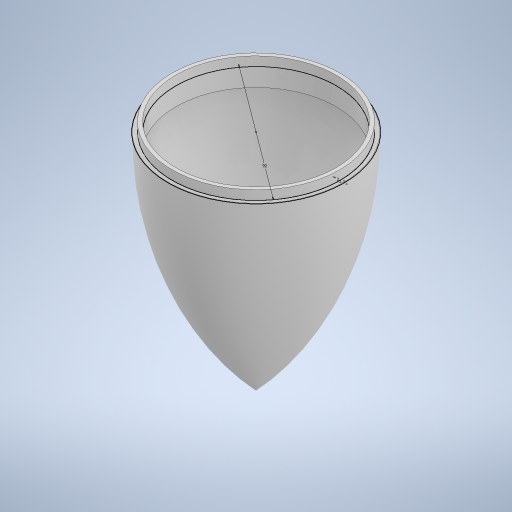
# Autodesk Inventor part: final탄두뚜껑1
Saved by Autodesk Inventor 2023 (Build 270158000, 158)
## iProperties
Created: 2023-10-31
Part Number: final탄두뚜껑1
Material: 일반
Document SubType Name: Modeling
Designer: rlatk
Density: 1 g/cm^3
Appearance: 기본값
Author: rlatk
Autodesk Inventor part; units mm, degrees
ref_plane "YZ Plane" through (0, 0, 0) normal (1, 0, 0) x (0, 1, 0)
ref_plane "XZ Plane" through (0, 0, 0) normal (0, 1, 0) x (-1, 0, 0)
ref_plane "XY Plane" through (0, 0, 0) normal (0, 0, 1) x (1, 0, 0)
sketch "스케치1" plane through (0, 0, 0) normal (0, 1, 0) x (-1, 0, 0)
  circle A0 centre (0, 0) radius 46
  circle A1 centre (0, 0) radius 44
  circle A2 centre (0, 0) radius 48.3
  dimension "d0" = 92
  dimension "d1" = 2
  dimension "d2" = 2.3
  constraints: 3 centre point, 1 coincident
  measures "d0" diameter of A0
  measures "d1" radial gap between concentric circles of A0 A1
  measures "d2" radial gap between concentric circles of A0 A2
extrude "돌출1" add sketch "스케치1" along normal blind 5 contours A0
sketch "스케치2" plane through (0, 0, 0) normal (0, 0, 1) x (1, 0, 0)
  line L0 (48.3, 0) -> (-48.3, 0) projected
  line L1 (46, 0) -> (-46, 0) projected
  arc A0 (-46, 0) -> (0, -120) centre (127.9848, -2.1225) ccw
  arc A1 (-48.0001, 0) -> (0, -122.9327) centre (127.9848, -2.1225) ccw
  line L2 (0, -122.9327) -> (0, -120)
  line L3 (-48.0001, 0) -> (-46, 0)
  line L4 (0, -154.1225) -> (0, 31.5204) projected
  point P0 (0, 0)
  point P1 (-48.0001, 0)
  dimension "d15" = 2
  constraints: 4 end point, 4 point on circle, 2 centre point, 1 horizontal
  measures "d15" radial gap between concentric circles of A0 A1
extrude "돌출3" add sketch "스케치1" against normal blind 10 contours A0
revolve "회전2" add sketch "스케치2" angle 360 about axis through (0, -10, 0) along (0, 1, 0) contours A0 L2 A1 L0
